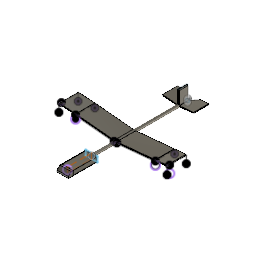
Final Plane Design (Autodesk Fusion 360 design; units mm, degrees)
Autodesk Fusion 360 part; units mm, degrees
sketch "Sketch1" plane through (0, 0, 0) normal (0, 0, 1) x (1, 0, 0)
  line L0 (0, 0) -> (18, 0)
  line L1 (18, 0) -> (18, 45)
  line L2 (18, 45) -> (0, 45)
  line L3 (0, 45) -> (0, 0)
  dimension "d1" = 18
  dimension "d2" = 45
  constraint horizontal L0
  constraint vertical L1
  constraint horizontal L2
  constraint vertical L3
  constraint coincident L0.start L3.end
  measures "d1" distance of L0.start L0.end
  measures "d2" distance of L0.start L2.end
extrude "Extrude1" add sketch "Sketch1" along normal blind 5 contours L0 L1 L2 L3 picked at (6, 30) makes body 1
copy_body "Body->Comp1" bodies 1 removing the originals makes body 2 in component "Component"
move_body "Move1" bodies 2 to x (1, 0, 0) y (0, 1, 0) z (0, 0, 1) at (0, 0, -2.5) in component "Component"
move_body "Move2" bodies 2 to x (1, 0, 0) y (0, 1, 0) z (0, 0, 1) at (-9, 0, 0) in component "Component"
sketch "blueprint" plane through (0, 0, 0) normal (0, 0, 1) x (1, 0, 0)
  line L0 (0, 45.000001) -> (0, 48.000001) construction
  line L1 (0, 48.000001) -> (12, 48.000001) construction
  line L2 (12, 48.000001) -> (12, -1.999999) construction
  line L3 (0, 48.000001) -> (3, 48.000001) construction
  line L4 (3, 48.000001) -> (3, 248.000001) construction
  line L5 (3, 248.000001) -> (0, 248.000001) construction
  line L6 (3, 248.000001) -> (15, 260) construction
  line L7 (3, 248.000001) -> (19.970562, 248.000001) construction
  line L8 (3, 248.000001) -> (3, 228.000001) construction
  line L9 (3, 228.000001) -> (33, 228.000001) construction
  line L10 (33, 228.000001) -> (33, 260) construction
  line L11 (33, 260) -> (15, 260) construction
  line L12 (3, 48.000001) -> (3, 98.000001) construction
  line L13 (3, 98.000001) -> (83, 98.000001) construction
  line L14 (83, 98.000001) -> (112.544233, 92.790555) construction
  line L15 (83, 98.000001) -> (113, 98.000001) construction
  line L16 (112.544233, 92.790555) -> (112.544233, 132.790555) construction
  line L17 (112.544233, 132.790555) -> (83, 138.000001) construction
  line L18 (83, 138.000001) -> (3, 138.000001) construction
  line L19 (83, 138.000001) -> (83, 98.000001) construction
  line L20 (0, 248.000001) -> (1.5, 248.000001)
  line L21 (0, 248.000001) -> (0, 228.000003) construction
  line L22 (0, 228.000003) -> (0.987502, 228.000003)
  line L23 (2, 228.000003) -> (1.974695, 229.012185) construction
  arc A0 (0.987502, 228.000003) -> (1.974695, 229.012185) centre (0.987502, 228.987505) ccw
  arc A1 (1.974695, 229.012185) -> (0, 228.987505) centre (0.987502, 228.987505) ccw construction
  arc A2 (0, 228.987505) -> (0.987502, 228.000003) centre (0.987502, 228.987505) ccw construction
  line L24 (-3, 98.000001) -> (-83, 98.000001) construction
  line L25 (0, 48.000001) -> (-12, 48.000001) construction
  line L26 (0, 45.000001) -> (0, 48.000001) construction
  line L27 (-83, 138.000001) -> (-83, 98.000001) construction
  line L28 (-112.544233, 132.790555) -> (-83, 138.000001) construction
  line L29 (-83, 98.000001) -> (-112.544233, 92.790555) construction
  line L30 (-12, 48.000001) -> (-12, -1.999999) construction
  line L31 (-83, 98.000001) -> (-113, 98.000001) construction
  line L32 (-83, 138.000001) -> (-3, 138.000001) construction
  line L33 (-112.544233, 92.790555) -> (-112.544233, 132.790555) construction
  line L34 (0, 248.000001) -> (-1.5, 248.000001)
  line L35 (-3, 48.000001) -> (-3, 98.000001) construction
  line L36 (0, 48.000001) -> (-3, 48.000001) construction
  line L37 (-33, 228.000001) -> (-33, 260) construction
  line L38 (-3, 248.000001) -> (-3, 228.000001) construction
  arc A3 (-0.987502, 228.000003) -> (0, 228.987505) centre (-0.987502, 228.987505) ccw construction
  line L39 (-0.987502, 228.000003) -> (-2, 228.000003) construction
  line L40 (-3, 248.000001) -> (0, 248.000001) construction
  line L41 (-33, 260) -> (-15, 260) construction
  line L42 (-1.974695, 229.012185) -> (-1.5, 248.000001)
  arc A4 (0, 228.987505) -> (-1.974695, 229.012185) centre (-0.987502, 228.987505) ccw construction
  line L43 (-3, 248.000001) -> (-15, 260) construction
  line L44 (-3, 48.000001) -> (-3, 248.000001) construction
  line L45 (-3, 228.000001) -> (-33, 228.000001) construction
  arc A5 (-1.974695, 229.012185) -> (-0.987502, 228.000003) centre (-0.987502, 228.987505) ccw
  line L46 (-3, 248.000001) -> (-19.970562, 248.000001) construction
  line L47 (-2, 228.000003) -> (-1.974695, 229.012185) construction
  line L48 (1.974695, 229.012185) -> (1.5, 248.000001)
  line L49 (0.987502, 228.000003) -> (2, 228.000003) construction
  line L50 (0, 228.000003) -> (-0.987502, 228.000003)
  point P0 (1, 228.000003)
  point P1 (1.972917, 229.083335)
  point P2 (-1.972917, 229.083335)
  point P3 (-1, 228.000003)
  dimension "d5" = 3
  dimension "d6" = 12
  dimension "d7" = 50
  dimension "d10" = 3
  dimension "d11" = 200
  dimension "d12" = 45
  dimension "d13" = 20
  dimension "d14" = 30
  dimension "d15" = 32
  dimension "d16" = 50
  dimension "d17" = 80
  dimension "d18" = 10
  dimension "d19" = 30
  dimension "d21" = 40
  dimension "d22" = 30
  dimension "d30" = 1.5
  dimension "d31" = 2
  dimension "d33" = 80
  constraint vertical L0
  constraint perpendicular L0 L1
  constraint perpendicular L1 L2
  constraint perpendicular L0 L3
  constraint perpendicular L1 L4
  constraint perpendicular L4 L5
  constraint horizontal L7
  constraint vertical L8
  constraint horizontal L9
  constraint perpendicular L9 L10
  constraint perpendicular L10 L11
  constraint vertical L12
  constraint horizontal L13
  constraint horizontal L15
  constraint perpendicular L4 L18
  constraint perpendicular L5 L21
  constraint perpendicular L8 L22
  constraint tangent L22 A0
  constraint tangent L21 A0
  constraint tangent L23 A0
  constraint concentric A0 A1
  constraint concentric A0 A2
  constraint parallel L14 L17
  constraint symmetric L6.end L21 L41.end
  constraint symmetric L10.end L21 L37.end
  constraint symmetric L21 A0 A5
  constraint symmetric L21 A1 A4
  constraint symmetric L21 A2 A3
  constraint tangent A0 L48
  constraint perpendicular L8 L49
  measures "d12" angle of L6 L7
  measures "d18" angle of L14 L15
extrude "Extrude21" add sketch "blueprint" along normal blind 30 separate body contours L20 L22 A0 L34 L42 A5 L48 L50 picked at (0, 235.341457) makes body 3
ref_plane "WorkPlane1" through (43, 98.000001, 0) normal (0, -1, 0) x (1, 0, 0)
ref_plane "WorkPlane2" through (83, 118.000001, 0) normal (-1, 0, 0) x (0, -1, 0)
ref_plane "WorkPlane3" through (112.544233, 112.790555, 0) normal (1, 0, 0) x (0, 1, 0)
sketch "Sketch4" plane through (112.544233, 112.790555, 0) normal (1, 0, 0) x (0, 1, 0)
  line L0 (-20, 0) -> (-20, 15) construction
  line L1 (20, 0) -> (20, 15) construction
  line L2 (-20, 15) -> (20, 15) construction
  point P0 (-20, 0)
  point P1 (20, 0)
  dimension "d26" = 15
  constraint coincident P0 L0.start
  constraint vertical L0
  constraint coincident P1 L1.start
  constraint vertical L1
  constraint equal L0 L1
  measures "d26" distance of P0 L0.end
sketch "midsec1" plane through (83, 118.000001, 0) normal (-1, 0, 0) x (0, -1, 0)
  line L0 (20, 0) -> (20, 7.5) construction
  line L1 (-20, 0) -> (-20, 7.5) construction
  line L2 (20, 7.5) -> (-20, 7.5) construction
  point P0 (20, 0)
  point P1 (-20, 0)
  dimension "d28" = 7.5
  constraint vertical L0
  constraint coincident P1 L1.start
  constraint vertical L1
  constraint equal L0 L1
  constraint perpendicular L1 L2
  measures "d28" distance of P0 L0.end
sketch "Front of Wing" plane through (43, 98.000001, 0) normal (0, -1, 0) x (1, 0, 0)
  line L0 (-40, 0) -> (40, 7.5)
  line L1 (40, 7.5) -> (69.544233, 15) construction
  point P0 (-40, 0)
  point P1 (40, 7.5)
  point P2 (69.544233, 15)
  point P3 (70, 0)
  point P4 (40, 0)
  constraint coincident P0 L0.start
  constraint coincident P1 L0.end
ref_plane "WorkPlane6" through (43, 98.000001, 3.75) normal (-0.093341, 0, 0.995634) x (0.995634, 0, 0.093341)
sketch "ws1" plane through (43, 98.000001, 3.75) normal (-0.093341, 0, 0.995634) x (0.995634, 0, 0.093341)
  line L0 (-40.175397, 150) -> (-28.227786, 162)
  line L1 (-10.30637, 162) -> (-28.227786, 162)
  line L2 (-10.30637, 130) -> (-10.30637, 162)
  line L3 (-40.175397, 130) -> (-10.30637, 130)
  line L4 (-40.175397, 150) -> (-40.175397, 130)
  line L5 (-40.175397, 40) -> (40.175397, 40)
  line L6 (40.175397, 40) -> (40.175397, 0)
  line L7 (40.175397, 0) -> (-40.175397, 0)
  line L8 (-40.175397, 0) -> (-40.175397, 40)
  point P0 (-40.175397, 130)
  point P1 (-40.175397, 150)
  point P2 (-40.175397, 150)
  point P3 (-40.175397, 130)
  point P4 (-10.30637, 130)
  point P5 (-10.30637, 162)
  point P6 (-28.227786, 162)
  point P7 (-40.175397, 40)
  point P8 (40.175397, 40)
  constraint perpendicular L5 L6
  constraint perpendicular L6 L7
  constraint perpendicular L5 L8
ref_plane "WorkPlane7" through (97.772116, 98.000001, 11.25) normal (0.246052, 0, -0.969257) x (0.969257, 0, 0.246052)
sketch "ws2" plane through (97.772116, 98.000001, 11.25) normal (0.246052, 0, -0.969257) x (0.969257, 0, 0.246052)
  line L0 (-15.240667, -40) -> (-15.240667, 0)
  line L1 (-15.240667, 0) -> (15.240667, 5.209445)
  line L2 (15.240667, 5.209445) -> (15.240667, -34.790555)
  line L3 (15.240667, -34.790555) -> (-15.240667, -40)
  point P0 (15.240667, -34.790555)
  point P1 (15.240667, 5.209445)
  point P2 (-15.240667, -40)
  point P3 (-15.240667, 0)
ref_plane "WorkPlane8" through (1.5, 248.000001, 0) normal (0, 1, 0) x (-1, 0, 0)
sketch "fuseoutline" plane through (1.5, 248.000001, 0) normal (0, 1, 0) x (1, 0, 0)
  line L0 (-1.5, 0) -> (-1.5, -3) construction
  line L1 (-1.5, 0) -> (-1.5, 3) construction
  circle A0 centre (-1.5, 0) radius 3
  constraint coincident L0.start L1.start
ref_plane "WorkPlane9" through (6, 48.000001, 0) normal (0, -1, 0) x (1, 0, 0)
sketch "back ard" plane through (6, 48.000001, 0) normal (0, -1, 0) x (1, 0, 0)
  circle A0 centre (-6, 0) radius 3.4
  circle A1 centre (-6, 0) radius 2.25
  line L0 (6, 5) -> (-18, 5)
  line L1 (-18, 5) -> (-18, -5)
  line L2 (-18, -5) -> (6, -5)
  line L3 (6, -5) -> (6, 5)
  line L4 (6, 5) -> (-18, -5) construction
  line L5 (-18, 5) -> (6, -5) construction
  line L6 (6, 5) -> (-18, 5)
  line L7 (-18, -5) -> (-18, 5)
  line L8 (-18, -5) -> (6, -5)
  line L9 (6, 5) -> (6, -5)
  point P0 (-6, 0)
  dimension "d42" = 4.5
  dimension "d43" = 10
  dimension "d44" = 24
  constraint concentric A0 A1
  constraint horizontal L0
  constraint perpendicular L0 L1
  constraint parallel L0 L2
  constraint parallel L1 L3
  constraint coincident L4 P0
  constraint coincident L5 P0
  constraint coincident P0 A0.centre
  measures "d42" diameter of A1
  measures "d43" distance of L0.end L1.end
  measures "d44" distance of L0.start L0.end
sketch "front triag1" plane through (0, 0, 0) normal (1, 0, 0) x (0, 1, 0)
  line L0 (48.000001, 5) -> (48.000001, -5) construction
  line L1 (48.000001, 5) -> (48.000001, -5) construction
  line L2 (48.000001, -5) -> (-1.999999, -5) construction
  line L3 (-1.999999, -5) -> (-1.999999, 5) construction
  line L4 (-1.999999, 5) -> (48.000001, 5) construction
  point P0 (-1.999999, 0)
  constraint perpendicular L1 L2
  constraint parallel L1 L3
  constraint parallel L2 L4
  constraint parallel L0 L1
ref_plane "WorkPlane10" through (18.352102, -1.999999, 0) normal (0, -1, 0) x (1, 0, 0)
sketch "front rec1" plane through (18.352102, -1.999999, 0) normal (0, -1, 0) x (1, 0, 0)
  line L0 (-6.352102, 5) -> (-30.352102, 5)
  line L1 (-30.352102, 5) -> (-30.352102, -5)
  line L2 (-30.352102, -5) -> (-6.352102, -5)
  line L3 (-6.352102, -5) -> (-6.352102, 5)
  line L4 (-30.352102, 5) -> (-6.352102, 5) construction
  line L5 (-6.352102, -5) -> (-6.352102, 5) construction
  line L6 (-30.352102, -5) -> (-30.352102, 5) construction
  line L7 (-6.352102, -5) -> (-30.352102, -5) construction
  line L8 (-7.352102, -4) -> (-7.352102, 4)
  line L9 (-29.352102, 4) -> (-7.352102, 4)
  line L10 (-29.352102, -4) -> (-29.352102, 4)
  line L11 (-7.352102, -4) -> (-29.352102, -4)
  point P0 (-30.352102, 0)
  point P1 (-6.352102, 0)
  point P2 (-18.352102, 0)
  point P3 (-18.352102, 5)
  point P4 (-18.352102, -5)
  point P5 (-30.352102, 5)
  point P6 (-6.352102, 5)
  point P7 (-6.352102, -5)
  point P8 (-30.352102, -5)
  dimension "d62" = -1
ref_plane "WorkPlane14" through (-83, 118.000001, 0) normal (-1, 0, 0) x (0, -1, 0)
sketch "left ws1" plane through (-83, 118.000001, 0) normal (-1, 0, 0) x (0, 1, 0)
  line L0 (-20, 0) -> (-20, -7.5) construction
  line L1 (20, 0) -> (20, -7.5) construction
  line L2 (-20, -7.5) -> (20, -7.5) construction
  point P0 (-20, 0)
  point P1 (20, 0)
  dimension "d51" = 7.5
  constraint coincident P0 L0.start
  constraint vertical L0
  constraint coincident P1 L1.start
  constraint vertical L1
  constraint equal L0 L1
  measures "d51" distance of P0 L0.end
ref_plane "WorkPlane15" through (-112.544233, 112.790555, 0) normal (1, 0, 0) x (0, 1, 0)
sketch "right ws2" plane through (-112.544233, 112.790555, 0) normal (1, 0, 0) x (0, 1, 0)
  line L0 (-20, 0) -> (-20, 15) construction
  line L1 (20, 0) -> (20, 15) construction
  line L2 (20, 15) -> (-20, 15) construction
  point P0 (-20, 0)
  point P1 (20, 0)
  dimension "d53" = 15
  constraint coincident P0 L0.start
  constraint vertical L0
  constraint coincident P1 L1.start
  constraint vertical L1
  constraint equal L0 L1
  measures "d53" distance of P0 L0.end
sketch "left side angled wings" plane through (43, 98.000001, 0) normal (0, -1, 0) x (1, 0, 0)
  line L0 (-46, 0) -> (-126, 7.5)
  line L1 (-126, 7.5) -> (-155.544233, 15) construction
  point P0 (-46, 0)
  point P1 (-126, 0)
  point P2 (-126, 7.5)
  point P3 (-155.544233, 15)
  constraint coincident P0 L0.start
  constraint coincident P2 L0.end
ref_plane "WorkPlane16" through (-43, 98.000001, 3.75) normal (0.093341, 0, 0.995634) x (-0.995634, 0, 0.093341)
sketch "Whole top ws1" plane through (-43, 98.000001, 3.75) normal (0.093341, 0, 0.995634) x (-0.995634, 0, 0.093341)
  line L0 (40, 0) -> (40, -40)
  line L1 (40, -40) -> (-40, -40)
  line L2 (-40, -40) -> (-40, 0)
  line L3 (-40, 0) -> (40, 0)
  line L4 (-10.30637, -130) -> (-10.30637, -162)
  line L5 (-40.175397, -130) -> (-10.30637, -130)
  line L6 (-40.175397, -150) -> (-40.175397, -130)
  line L7 (-40.175397, -150) -> (-28.227786, -162)
  line L8 (-10.30637, -162) -> (-28.227786, -162)
  point P0 (-10.30637, -162)
  point P1 (-10.30637, -130)
  constraint vertical L0
  constraint perpendicular L0 L1
  constraint perpendicular L1 L2
  constraint perpendicular L0 L3
ref_plane "WorkPlane17" through (-97.772116, 98.000001, 11.25) normal (-0.246052, 0, -0.969257) x (-0.969257, 0, 0.246052)
sketch "Sketch22" plane through (-97.772116, 98.000001, 11.25) normal (-0.246052, 0, -0.969257) x (-0.969257, 0, 0.246052)
  line L0 (15.240667, 34.790555) -> (15.240667, -5.209445)
  line L1 (15.240667, -5.209445) -> (-15, 0)
  line L2 (-15, 0) -> (-15, 40)
  line L3 (-15, 40) -> (15.240667, 34.790555)
  point P0 (15.240667, 34.790555)
  point P1 (15.240667, -5.209445)
  constraint parallel L0 L2
  constraint parallel L1 L3
extrude "Extrude2" add sketch "back ard" against normal blind 130 separate body contours A0 picked at (-3.004369, -0.280696) makes body 4
sketch "Sketch23" plane through (0, 0, 0) normal (0, 0, 1) x (1, 0, 0)
sketch "fuse shell end" plane through (0, 178.000001, 0) normal (0, 1, 0) x (-1, 0, 0)
  circle A0 centre (0, 0) radius 2.25
  circle A1 centre (0, 0) radius 3.4
  circle A2 centre (0, 0) radius 3
  constraint concentric A0 A2
extrude "Extrude3" add sketch "fuse shell end" along normal blind 70 contours A0 | A1 | A2 picked at (1.155625, -0.747903) picked at (3.254008, -0.168915) picked at (2.730454, -0.260824) bodies 4
surface "SurfacePatch1" add patch profiles "back ard" section 1 contours L0 L1 L2 L3 L6 L7 L8 L9 picked at (3.133333, 0) separate body makes body 5
extrude "Extrude4" add sketch "back ard" along normal blind 50 separate body contours L0 L1 L2 L3 L6 L7 L8 L9 picked at (3.133333, 0) makes body 6
extrude "Extrude5" cut sketch "front rec1" against normal blind 49 contours L8 L9 L10 L11 picked at (-14.685435, -1.333333) bodies 6
extrude "Extrude6" add sketch "Whole top ws1" along normal blind 2 separate body contours L4 L5 L6 L7 L8 picked at (-30.219054, -136.666667) makes body 7
extrude "Extrude7" add sketch "ws1" along normal blind 2 separate body contours L0 L1 L2 L3 L4 picked at (-30.219054, 136.666667) makes body 8
extrude "Extrude8" add sketch "back ard" along normal blind 1.5 contours A0 picked at (-3.004369, -0.280696) bodies 4 6
extrude "Extrude9" cut 1 faces at (2.995631, 46.500001, -0.280696) along direction (0, 1, 0) blind 1.5 on bodies 4 bodies 4
extrude "Extrude10" add sketch "back ard" along normal blind 2.5 contours A0 picked at (-3.004369, -0.280696) bodies 4
extrude "Extrude11" cut 1 faces at (2.995631, 45.500001, -0.280696) along direction (0, 1, 0) blind 0.5 on bodies 4 bodies 4
sketch "right wing top" plane through (43, 98.000001, 3.75) normal (-0.093341, 0, 0.995634) x (0.995634, 0, 0.093341)
  line L0 (40, 40) -> (-40.000001, 40)
  line L1 (-40.000001, 40) -> (-40.000001, 0)
  line L2 (40, 40) -> (-40.000001, 40)
  line L3 (-40.000001, 40) -> (-40.000001, 0)
  line L4 (40, 0) -> (-40.000001, 0)
  line L5 (40, 0) -> (40, 40)
  constraint horizontal L0
  constraint perpendicular L0 L1
  constraint perpendicular L3 L4
  constraint perpendicular L0 L5
sketch "left wing top" plane through (-43, 98.000001, 3.75) normal (0.093341, 0, 0.995634) x (-0.995634, 0, 0.093341)
  line L0 (40, -40) -> (-40, -40)
  line L1 (-40, -40) -> (-40, 0)
  line L2 (-40, 0) -> (40, 0)
  line L3 (40, 0) -> (40, -40)
  constraint horizontal L0
  constraint perpendicular L0 L1
  constraint perpendicular L1 L2
  constraint perpendicular L0 L3
extrude "Extrude12" add sketch "Sketch22" against normal blind 2 separate body contours L0 L1 L2 L3 picked at (5.160444, 9.86037) makes body 9
extrude "Extrude13" add sketch "left wing top" along normal blind 2 separate body contours L0 L1 L2 L3 picked at (13.333333, -26.666667) makes body 10
extrude "Extrude14" add 1 faces at (-82.763142, 111.333334, 8.147384) along direction (-0.99563423, 0, 0.09334071) blind 0.2 on bodies 10 bodies 10 9
extrude "Extrude15" add 1 faces at (-83.006949, 124.666667, 8.450739) along direction (0.96925657, 0, -0.24605223) blind 0.3 on bodies 10 bodies 10
extrude "Extrude16" add 1 faces at (-3.112404, 124.666667, 0.680128) along direction (0.99563423, 0, -0.09334071) blind 0.3 separate body on bodies 10 makes body 11
combine "Combine1" operation add target body 11 tool bodies 10
copy_body "Body->Comp2" bodies 11 removing the originals makes body 12 in component "left wing"
extrude "Extrude17" add sketch "ws2" against normal blind 2 separate body contours L0 L1 L2 L3 picked at (5.080222, -9.86037) makes body 13
extrude "Extrude18" add sketch "right wing top" along normal blind 2 separate body contours L0 L1 L2 L3 L4 L5 picked at (-13.333334, 26.666667) makes body 14
extrude "Extrude19" add 1 faces at (3.112403, 124.666667, 0.680128) along direction (-0.99563423, 0, -0.09334071) blind 0.5 separate body on bodies 14 makes body 15
combine "Combine2" operation add target body 13 tool bodies 14 15
copy_body "Body->Comp3" bodies 13 removing the originals makes body 16 in component "right wing"
sketch "Sketch2" plane through (0, -1.999999, 0) normal (0, -1, 0) x (1, 0, 0) in component "case pyramid"
  line L0 (-11, 4) -> (11, 4)
  line L1 (11, 4) -> (11, -4)
  line L2 (11, -4) -> (-11, -4)
  line L3 (-11, -4) -> (-11, 4)
  line L4 (-12, -5) -> (12, -5)
  line L5 (12, -5) -> (12, 5)
  line L6 (12, 5) -> (-12, 5)
  line L7 (-12, 5) -> (-12, -5)
  line L8 (-12, 5) -> (12, 5)
  line L9 (12, 5) -> (12, -5)
  line L10 (12, -5) -> (-12, -5)
  line L11 (-12, -5) -> (-12, 5)
  line L12 (-11, 4) -> (11, 4)
  line L13 (11, 4) -> (11, -4)
  line L14 (11, -4) -> (-11, -4)
  line L15 (-11, -4) -> (-11, 4)
  constraint horizontal L8
  constraint vertical L9
  constraint horizontal L10
  constraint vertical L11
  constraint coincident L4.end L5.start
  constraint coincident L6.end L7.start
  constraint horizontal L12
  constraint vertical L13
  constraint horizontal L14
  constraint vertical L15
  constraint coincident L1.end L2.start
  constraint coincident L0.start L3.end
sketch "Sketch3" plane through (0, 0, 0) normal (0, 0, 1) x (1, 0, 0) in component "case pyramid"
extrude "Extrude1'" add sketch "Sketch2" along normal blind 10 separate body contours L0 L1 L2 L3 L12 L13 L14 L15 | L4 L5 L6 L7 L8 L9 L10 L11 picked at (-3.666667, -1.333333) picked at (-3.666667, -4.666667) makes body 17 in component "case pyramid"
sketch "Sketch29" plane through (0, -1.999999, 0) normal (0, -1, 0) x (1, 0, 0)
chamfer "Chamfer1" distance 6 angle 45 1 edges at (0, -11.999999, 5) on bodies 17 in component "case pyramid"
shell "Shell1" thickness 2 removed faces 1 at (-4, -1.999999, 1.666667) on bodies 17 in component "case pyramid"
sketch "Sketch30" plane through (0, 0, 0) normal (0, 0, 1) x (1, 0, 0)
  circle A0 centre (0, 114.000002) radius 2
extrude "Extrude20" cut sketch "Sketch30" against normal blind 4 contours A0 picked at (1.037947, 114.375548) bodies 4
sketch "Sketch31" plane through (0, 0, 30) normal (0, 0, 1) x (-1, 0, 0)
  arc A0 (-0.987502, -228.000003) -> (-1.974695, -229.012185) centre (-0.987502, -228.987505) ccw
  line L0 (-1.974695, -229.012185) -> (-1.5, -248.000001)
  line L1 (-1.5, -248.000001) -> (1.5, -248.000001)
  line L2 (1.5, -248.000001) -> (1.974695, -229.012185)
  arc A1 (1.974695, -229.012185) -> (0.987502, -228.000003) centre (0.987502, -228.987505) ccw
  line L3 (0.987502, -228.000003) -> (-0.987502, -228.000003)
  line L4 (0, -228.000003) -> (0, -248.000001) construction
fillet "Fillet1" radius 1.5 1 faces at (0, 235.341457, 30) on bodies 3
ref_plane "WorkPlane11" through (0, 48.000001, 0) normal (-0.384615, 0, 0.923077) x (-0.923077, 0, -0.384615)
sketch "front diag1" plane through (0, 48.000001, 0) normal (-0.384615, 0, 0.923077) x (-0.923077, 0, -0.384615)
  line L0 (13, 50) -> (0, 56.928203)
  line L1 (0, 56.928203) -> (-13, 50)
  point P0 (13, 50)
  point P1 (-13, 50)
  point P2 (0, 56.928203)
  constraint coincident P0 L0.start
  constraint coincident P1 L1.end
component "Component" placed x (1, 0, 0) y (0, 1, 0) z (0, 0, 1) at (0, 0, 0)
component "case pyramid" placed x (1, 0, 0) y (0, 1, 0) z (0, 0, 1) at (0, 0, 0)
component "left wing" placed x (1, 0, 0) y (0, 1, 0) z (0, 0, 1) at (0, 0, 0)
component "right wing" placed x (1, 0, 0) y (0, 1, 0) z (0, 0, 1) at (0, 0, 0)
named bodies: "Arduino", "fuselage", "rectangle", "brains/arduino case", "left hors stab", "right hors stab", "left wing", "right wing"
